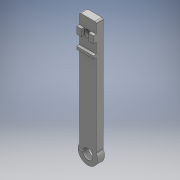
# Autodesk Inventor part: filament guide
Saved by Autodesk Inventor 2016 (Build 200138000, 138)
## iProperties
Created: 2016-03-07
Part Number: filament guide
Material: Generic
Document SubType Name: Modeling
Designer: Erwin
Density: 1 g/cm^3
Appearance: Default
Author: Erwin
Autodesk Inventor part; units mm, degrees
ref_plane "YZ Plane" through (0, 0, 0) normal (1, 0, 0) x (0, 1, 0)
ref_plane "XZ Plane" through (0, 0, 0) normal (0, 1, 0) x (-1, 0, 0)
ref_plane "XY Plane" through (0, 0, 0) normal (0, 0, 1) x (1, 0, 0)
sketch "Sketch1" plane through (0, 0, 0) normal (0, 1, 0) x (-1, 0, 0)
  circle A0 centre (0, 0) radius 5
  line L0 (-6, 85) -> (6, 85)
  arc A1 (-6, 3.6056) -> (6, 3.6056) centre (0, 0) ccw
  line L1 (-6, 3.6056) -> (-6, 85)
  line L2 (6, 85) -> (6, 3.6056)
  point P0 (-6, 0)
  point P1 (-5, 85)
  point P2 (5, 85)
  constraints: 6 end point, 3 point on line, 2 centre point, 2 point on circle, 1 coincident, 1 parallel
extrude "Extrusion1" add sketch "Sketch1" along normal blind 5
sketch "Sketch2" plane through (0, 5, 0) normal (0, 1, 0) x (1, 0, 0)
  line L0 (-6, -85) -> (6, -85) construction
  line L1 (0, -85) -> (0, -75) construction
  point P0 (0, 0)
  point P1 (-5, -85)
  point P2 (5, -85)
  dimension "d5" = 10
  constraints: 2 end point, 1 midpoint, 1 vertical
  measures "d5" distance of L1.start L1.end
hole "Hole1" at (0, 5, 75) direction (0, -1, 0) diameter 5.1 end through all
draft "FaceDraft1" angle 15 pull direction (0, 1, 0) faces at (-4.9353, 3.3333, -0.8021) fixed edges at (5, 5, 0)
sketch "Sketch3" plane through (0, 0, 0) normal (0, -1, 0) x (1, 0, 0)
  line L0 (0, 0) -> (-10, 0)
  line L1 (-10, 0) -> (-10, 0.6)
  line L2 (-10, 0.6) -> (0, 0.6)
  line L3 (0, 0.6) -> (0, 0)
  dimension "d15" = 0.6
  dimension "d19" = 10
  constraints: 8 end point, 2 parallel, 1 horizontal, 1 perpendicular
  measures "d15" distance of L0.end L1.end
  measures "d19" distance between parallel lines of L1 L3
extrude "Extrusion2" cut sketch "Sketch3" against normal blind 10
fillet "Fillet2" radius 0.5 2 edges at (-4.2347, 2.3015, 0.6) (-4.3301, 2.5, 0)
sketch "Sketch4" plane through (0, 0, 0) normal (0, -1, 0) x (1, 0, 0)
  line L0 (6, 85) -> (-6, 85) construction
  line L1 (0, 85) -> (0, 65) construction
  line L2 (5, 84) -> (5, 4.3589) projected
  line L3 (-5, 4.3589) -> (-5, 84) projected
  line L4 (5, 65) -> (-5, 65)
  line L5 (-5, 65) -> (-5, 63)
  line L6 (-5, 63) -> (5, 63)
  line L7 (5, 63) -> (5, 65)
  line L8 (-5, 77.5) -> (5, 77.5)
  line L9 (5, 77.5) -> (5, 72.5)
  line L10 (5, 72.5) -> (-5, 72.5)
  line L11 (-5, 72.5) -> (-5, 77.5)
  line L12 (-5, 77.5) -> (5, 72.5) construction
  line L13 (5, 77.5) -> (-5, 72.5) construction
  circle A0 centre (0, 75) radius 2.55 projected
  point P0 (0, 0)
  point P1 (4, 85)
  point P2 (-4, 85)
  dimension "d21" = 20
  dimension "d22" = 2
  dimension "d23" = 5
  constraints: 22 end point, 4 midpoint, 4 parallel, 3 point on line, 2 horizontal, 2 perpendicular, 1 vertical
  measures "d21" distance of L1.start L1.end
  measures "d22" distance of L5.end L4.end
  measures "d23" distance of L8.end L9.end
extrude "Extrusion3" add sketch "Sketch4" along normal blind 2 contours L2 L10 A0 L8 | L2 L6 L3 L4 | A0 L10 L3 L8
sketch "Sketch5" plane through (0, -2, 0) normal (0, -1, 0) x (1, 0, 0)
  arc A0 (0.5025, 72.5) -> (0.5025, 77.5) centre (0, 75) ccw projected
  circle A1 centre (0, 75) radius 2.55 projected
  line L0 (2.55, 77.55) -> (-2.55, 77.55)
  line L1 (-2.55, 77.55) -> (-2.55, 72.45)
  line L2 (-2.55, 72.45) -> (2.55, 72.45)
  line L3 (2.55, 72.45) -> (2.55, 77.55)
  line L4 (2.55, 77.55) -> (-2.55, 72.45) construction
  line L5 (-2.55, 77.55) -> (2.55, 72.45) construction
  arc A2 (-0.5025, 72.5) -> (0.5025, 72.5) centre (0, 75) ccw projected
  arc A3 (0.5025, 77.5) -> (-0.5025, 77.5) centre (0, 75) ccw projected
  arc A4 (-0.5025, 77.5) -> (-0.5025, 72.5) centre (0, 75) ccw projected
  point P0 (0, 0)
  dimension "d26" = 5.1
  dimension "d27" = 5.1
  constraints: 12 end point, 2 midpoint, 2 parallel, 1 horizontal, 1 perpendicular
  measures "d26" distance of L2.end L1.end
  measures "d27" distance of L1.end L0.end
extrude "Extrusion4" cut sketch "Sketch5" against normal blind 2 contours A0 L3 L2 A1 | A0 A1 L0 L3 | L2 L1 A1 | A1 L1 L0
sketch "Sketch6" plane through (-5, 0, 72.5) normal (-1, 0, 0) x (0, 0, 1)
  line L0 (0, 0) -> (5, 0) projected
  line L1 (0, 0) -> (0, -2) projected
  line L2 (5, -2) -> (0, -2) projected
  line L3 (5, 0) -> (5, -2) projected
  line L4 (-9.5, 0) -> (-7.5, 0) projected
  line L5 (-9.5, 0) -> (-9.5, -2) projected
  line L6 (-7.5, -2) -> (-9.5, -2) projected
  line L7 (-7.5, 0) -> (-7.5, -2) projected
  point P0 (-72.5, 0)
extrude "Extrusion5" add sketch "Sketch6" along normal blind 1
sketch "Sketch7" plane through (5, 0, 77.5) normal (1, 0, 0) x (0, 0, -1)
  line L0 (0, 0) -> (5, 0) projected
  line L1 (0, 0) -> (0, -2) projected
  line L2 (5, -2) -> (0, -2) projected
  line L3 (5, 0) -> (5, -2) projected
  line L4 (12.5, 0) -> (14.5, 0) projected
  line L5 (12.5, 0) -> (12.5, -2) projected
  line L6 (14.5, -2) -> (12.5, -2) projected
  line L7 (14.5, 0) -> (14.5, -2) projected
  point P0 (77.5, 0)
extrude "Extrusion6" add sketch "Sketch7" along normal blind 1
fillet "Fillet4" radius 1 4 edges at (6, 2.5, 85) (-6, 2.5, 85) (6, 2.5, 3.6056) (-6, 2.5, 3.6056)
body "Solid1"
